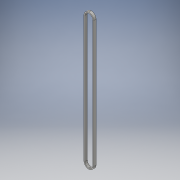
# Autodesk Inventor part: LiftWireLine14in
Saved by Autodesk Inventor 2016 (Build 200138000, 138)
## iProperties
Created: 2016-12-21
Part Number: LiftWireLine14in
Material: Generic
Document SubType Name: Modeling
Designer: RoboticsUser
Density: 1 g/cm^3
Appearance: Default
Author: RoboticsUser
Autodesk Inventor part; units mm, degrees
ref_plane "YZ Plane" through (0, 0, 0) normal (1, 0, 0) x (0, 1, 0)
ref_plane "XZ Plane" through (0, 0, 0) normal (0, 1, 0) x (-1, 0, 0)
ref_plane "XY Plane" through (0, 0, 0) normal (0, 0, 1) x (1, 0, 0)
sketch "Sketch1" plane through (0, 0, 0) normal (0, 0, 1) x (1, 0, 0)
  line L0 (0, 0) -> (25.4094, 0)
  line L1 (25.4094, 0) -> (25.4094, -355.6)
  line L2 (25.4094, -355.6) -> (0, -355.6)
  line L3 (0, -355.6) -> (0, 0)
  dimension "d0" = 355.6
  constraints: 8 end point, 2 parallel, 1 horizontal, 1 perpendicular
  measures "d0" distance of L0.end L1.end
extrude "Extrusion1" add sketch "Sketch1" along normal blind 6.35
fillet "Fillet1" radius 12.7 1 edges at (0, 0, 3.175)
fillet "Fillet2" radius 12.7 1 edges at (25.4094, 0, 3.175)
fillet "Fillet3" radius 12.7 1 edges at (25.4094, -355.6, 3.175)
fillet "Fillet4" radius 12.7 1 edges at (0, -355.6, 3.175)
shell "Shell1" thickness 2.54 removed faces 1 at (8.4698, -122.7667, 0)
shell "Shell2" thickness 2.54 removed faces 2 at (9.3165, -122.7667, 3.81) at (8.4698, -122.7667, 6.35)
body "Solid1"
